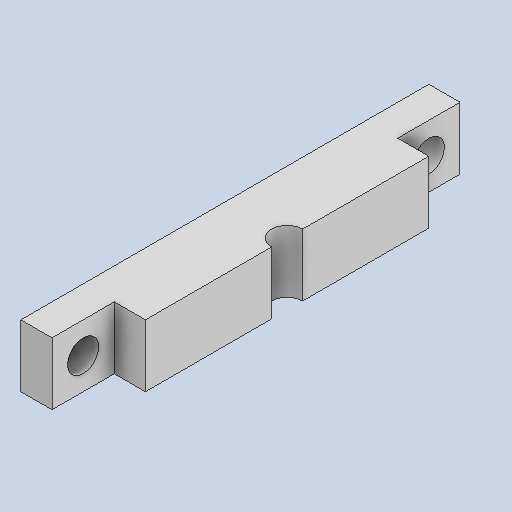
# Autodesk Inventor part: SoporteTubosSuperior_CPY
Saved by Autodesk Inventor 2023 (Build 270158000, 158)
## iProperties
Created: 2023-04-07
Part Number: SoporteTubosSuperior_CPY
Material: Generic
Document SubType Name: Modeling
Designer: Lenovo
Density: 1 g/cm^3
Appearance: Default
Author: Lenovo
Autodesk Inventor part; units mm, degrees
ref_plane "YZ Plane" through (0, 0, 0) normal (1, 0, 0) x (0, 1, 0)
ref_plane "XZ Plane" through (0, 0, 0) normal (0, 1, 0) x (-1, 0, 0)
ref_plane "XY Plane" through (0, 0, 0) normal (0, 0, 1) x (1, 0, 0)
sketch "Sketch1" plane through (0, 0, 0) normal (1, 0, 0) x (0, 1, 0)
  line L0 (-6, -12.5) -> (-6, -12.9)
  arc A0 (-6, -12.9) -> (-5.6, -13.3) centre (-5.6, -12.9) ccw
  line L1 (-5.6, -13.3) -> (-4.9, -13.3)
  arc A1 (-4.9, -13.3) -> (-4.7, -13.1) centre (-4.9, -13.1) ccw
  line L2 (-4.7, -13.1) -> (-4.7, -12.85)
  arc A2 (-4.5, -12.65) -> (-4.7, -12.85) centre (-4.5, -12.85) ccw
  line L3 (-4.5, -12.65) -> (-1.8, -12.65)
  arc A3 (-1.4, -13.05) -> (-1.8, -12.65) centre (-1.8, -13.05) ccw
  line L4 (-1.4, -13.05) -> (-1.4, -18.75)
  line L5 (-1.8, -19.15) -> (-4.5, -19.15)
  arc A4 (-1.8, -19.15) -> (-1.4, -18.75) centre (-1.8, -18.75) ccw
  arc A5 (-4.7, -18.95) -> (-4.5, -19.15) centre (-4.5, -18.95) ccw
  line L6 (-4.7, -18.95) -> (-4.7, -18.7)
  arc A6 (-4.7, -18.7) -> (-4.9, -18.5) centre (-4.9, -18.7) ccw
  line L7 (-4.9, -18.5) -> (-5.6, -18.5)
  arc A7 (-5.6, -18.5) -> (-6, -18.9) centre (-5.6, -18.9) ccw
  line L8 (-6, -18.9) -> (-6, -19.5)
  line L9 (-6.5, -6.5) -> (-6.5, -12.5)
  line L10 (-6.5, -12.5) -> (-2.5, -12.5)
  line L11 (-1.05, -19.5) -> (-6.5, -19.5)
  line L12 (-6.5, -19.5) -> (-6.5, -26)
  line L13 (-6.5, -26) -> (-1.05, -26)
  line L14 (-6, -26) -> (-6, -26.6)
  arc A8 (-6, -26.6) -> (-5.6, -27) centre (-5.6, -26.6) ccw
  line L15 (-5.6, -27) -> (-4.9, -27)
  arc A9 (-4.9, -27) -> (-4.7, -26.8) centre (-4.9, -26.8) ccw
  arc A10 (-4.5, -26.35) -> (-4.7, -26.55) centre (-4.5, -26.55) ccw
  line L16 (-4.7, -26.8) -> (-4.7, -26.55)
  line L17 (-4.5, -26.35) -> (-1.8, -26.35)
  arc A11 (-1.4, -26.75) -> (-1.8, -26.35) centre (-1.8, -26.75) ccw
  line L18 (-1.4, -26.75) -> (-1.4, -32.45)
  arc A12 (-1.8, -32.85) -> (-1.4, -32.45) centre (-1.8, -32.45) ccw
  line L19 (-1.8, -32.85) -> (-4.5, -32.85)
  arc A13 (-4.7, -32.65) -> (-4.5, -32.85) centre (-4.5, -32.65) ccw
  line L20 (-4.7, -32.65) -> (-4.7, -32.4)
  arc A14 (-4.7, -32.4) -> (-4.9, -32.2) centre (-4.9, -32.4) ccw
  line L21 (-4.9, -32.2) -> (-5.6, -32.2)
  arc A15 (-5.6, -32.2) -> (-6, -32.6) centre (-5.6, -32.6) ccw
  line L22 (-6, -32.6) -> (-6, -33)
  line L23 (-2.5, -33) -> (-6.5, -33)
  line L24 (-6.5, -33) -> (-6.5, -39)
  line L25 (32.5, 0) -> (0, 0)
  circle A16 centre (0, -6.5) radius 4.75
  circle A17 centre (32.5, -6.5) radius 4.75
  circle A18 centre (0, -39) radius 4.75
  circle A19 centre (32.5, -39) radius 4.75
  line L26 (39, -26) -> (39, -19.5)
  line L27 (39, -12.5) -> (39, -6.5)
  line L28 (39, -39) -> (39, -33)
  line L29 (26.5, -45.5) -> (32.5, -45.5)
  line L30 (0, -45.5) -> (6, -45.5)
  line L31 (13, -45.5) -> (19.5, -45.5)
  circle A20 centre (16.25, -22.75) radius 15
  circle A21 centre (16.2588, 5.0016) radius 2.5
  circle A22 centre (16.25, -50.5) radius 2.5
  circle A23 centre (16.25, -22.75) radius 5
  circle A24 centre (16.25, -22.75) radius 8.45
  line L32 (24.75, -27.6575) -> (24.75, -17.8425)
  line L33 (44, 10) -> (-11.5, 10)
  line L34 (-11.5, 10) -> (-11.5, -55.5)
  line L35 (-11.5, -55.5) -> (44, -55.5)
  line L36 (44, -55.5) -> (44, 10)
  line L37 (-11.5, 30) -> (44, 30)
  line L38 (-11.5, -75.5) -> (-11.5, 30)
  line L39 (44, 30) -> (44, -75.5)
  line L40 (44, -75.5) -> (-11.5, -75.5)
  circle A25 centre (16.25, -65.5) radius 5
  circle A26 centre (16.25, 20) radius 5
  arc A27 (11.25, -55.5) -> (21.25, -55.5) centre (16.25, -55.5) ccw
  line L41 (21.25, 10) -> (21.25, -55.5)
  line L42 (11.25, -55.5) -> (11.25, 10)
  arc A28 (21.25, 10) -> (11.25, 10) centre (16.25, 10) ccw
  line L43 (21.25, -45.5) -> (11.25, -45.5)
  point P0 (21.25, 0)
  point P1 (11.25, 0)
  constraints: 88 end point, 36 point on circle, 29 centre point, 6 point on line, 5 horizontal, 4 vertical, 2 midpoint, 16 other
extrude "Extrusion1" add sketch "Sketch1" along normal blind 10 contours L41 A20 L42 L25 | L41 A24 L42 A20 | L41 A23 L42 A24 | L42 A24 L41 A20 | A20 L41 L43 L31 L42 | A23 | L41 A24 L42 A23
extrude "Extrusion2" add sketch "Sketch1" along normal blind 5 contours L25 L42 L33 L41 | L43 L31 L41 L35 L42
sketch "Sketch4" plane through (10, 21.25, 0) normal (0, 1, 0) x (1, 0, 0)
  line L0 (0, 45.5) -> (0, 0) projected
  circle A0 centre (0, 22.75) radius 2.5
  point P0 (-10, 0)
  dimension "d7" = 5
  constraints: 1 centre point, 1 midpoint
  measures "d7" diameter of A0
extrude "Extrusion4" cut sketch "Sketch4" against normal blind 10
body "Solid1"
